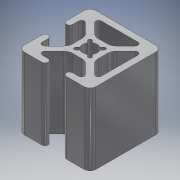
# Autodesk Inventor part: 1002-S
Saved by Autodesk Inventor 2017 SP1 (Build 210196100, 196)
## iProperties
Created: 2016-09-13
Part Number: 1002-S
Material: 6105-T5
Description: 40 S SHORT SINGLE UNIBEARING ASSEMBLY ON 40-4040 X 75mm
Document SubType Name: Modeling
Designer: BRALEF
Density: 1 g/cm^3
Appearance: CLEAR ANODIZED
MATERIAL: 6061-T6
PART PRICE: 44.65
Author: BRALEF
Autodesk Inventor part; units mm, degrees
ref_plane "YZ Plane" through (0, 0, 0) normal (1, 0, 0) x (0, 1, 0)
ref_plane "XZ Plane" through (0, 0, 0) normal (0, 1, 0) x (-1, 0, 0)
ref_plane "XY Plane" through (0, 0, 0) normal (0, 0, 1) x (1, 0, 0)
sketch "Sketch1" plane through (0, 0, 0) normal (0, 1, 0) x (-1, 0, 0)
  arc A0 (-1.9692, 2.8605) -> (-2.8605, 1.9692) centre (-2.4696, 2.4696) ccw
  line L0 (-2.2319, 1.3405) -> (-2.8605, 1.9692)
  arc A1 (-2.2319, 1.3405) -> (-2.2319, -1.3405) centre (0, 0) ccw
  line L1 (-2.8605, -1.9692) -> (-2.2319, -1.3405)
  arc A2 (-2.8605, -1.9692) -> (-1.9692, -2.8605) centre (-2.4696, -2.4696) ccw
  line L2 (-1.3405, -2.2319) -> (-1.9692, -2.8605)
  arc A3 (-1.3405, -2.2319) -> (1.3405, -2.2319) centre (0, 0) ccw
  line L3 (1.9692, -2.8605) -> (1.3405, -2.2319)
  arc A4 (1.9692, -2.8605) -> (2.8605, -1.9692) centre (2.4696, -2.4696) ccw
  line L4 (2.2319, -1.3405) -> (2.8605, -1.9692)
  arc A5 (2.2319, -1.3405) -> (2.2319, 1.3405) centre (0, 0) ccw
  line L5 (2.8605, 1.9692) -> (2.2319, 1.3405)
  arc A6 (2.8605, 1.9692) -> (1.9692, 2.8605) centre (2.4696, 2.4696) ccw
  line L6 (1.3405, 2.2319) -> (1.9692, 2.8605)
  arc A7 (1.3405, 2.2319) -> (-1.3405, 2.2319) centre (0, 0) ccw
  line L7 (-1.9692, 2.8605) -> (-1.3405, 2.2319)
  arc A8 (-8.7558, 7.1932) -> (-10.4902, 6.4748) centre (-9.4742, 6.4748) ccw
  line L8 (-10.4902, -6.4748) -> (-10.4902, 6.4748)
  arc A9 (-10.4902, -6.4748) -> (-8.7558, -7.1932) centre (-9.4742, -6.4748) ccw
  line L9 (-5.4471, -3.8845) -> (-8.7558, -7.1932)
  arc A10 (-5.4471, -3.8845) -> (-4.5172, -1.6395) centre (-7.6922, -1.6395) ccw
  line L10 (-4.5172, 1.6395) -> (-4.5172, -1.6395)
  arc A11 (-4.5172, 1.6395) -> (-5.4471, 3.8845) centre (-7.6922, 1.6395) ccw
  line L11 (-8.7558, 7.1932) -> (-5.4471, 3.8845)
  arc A12 (3.8845, -5.4471) -> (1.6395, -4.5172) centre (1.6395, -7.6922) ccw
  line L12 (-1.6395, -4.5172) -> (1.6395, -4.5172)
  arc A13 (-1.6395, -4.5172) -> (-3.8845, -5.4471) centre (-1.6395, -7.6922) ccw
  line L13 (-7.1932, -8.7558) -> (-3.8845, -5.4471)
  arc A14 (-7.1932, -8.7558) -> (-6.4748, -10.4902) centre (-6.4748, -9.4742) ccw
  line L14 (6.4748, -10.4902) -> (-6.4748, -10.4902)
  arc A15 (6.4748, -10.4902) -> (7.1932, -8.7558) centre (6.4748, -9.4742) ccw
  line L15 (3.8845, -5.4471) -> (7.1932, -8.7558)
  arc A16 (-12.7002, -10.5921) -> (-10.592, -12.7003) centre (-10.592, -10.5921) ccw
  line L16 (-12.7002, -10.5921) -> (-12.7002, 10.5915)
  arc A17 (-10.592, 12.6997) -> (-12.7002, 10.5915) centre (-10.592, 10.5915) ccw
  line L17 (-10.592, 12.6997) -> (-4.3561, 12.6997)
  arc A18 (-4.3561, 10.4899) -> (-4.3561, 12.6997) centre (-4.3561, 11.5948) ccw
  line L18 (-4.3561, 10.4899) -> (-6.4746, 10.4899)
  arc A19 (-6.4746, 10.4899) -> (-7.193, 8.7555) centre (-6.4746, 9.4739) ccw
  line L19 (-7.193, 8.7555) -> (-3.8847, 5.4472)
  arc A20 (-3.8847, 5.4472) -> (-1.6396, 4.5172) centre (-1.6396, 7.6922) ccw
  line L20 (-1.6396, 4.5172) -> (1.6395, 4.5172)
  arc A21 (1.6395, 4.5172) -> (3.8846, 5.4472) centre (1.6395, 7.6922) ccw
  line L21 (3.8846, 5.4472) -> (7.1929, 8.7555)
  arc A22 (7.1929, 8.7555) -> (6.4745, 10.4899) centre (6.4745, 9.4739) ccw
  line L22 (6.4745, 10.4899) -> (4.3561, 10.4899)
  arc A23 (4.3561, 12.6997) -> (4.3561, 10.4899) centre (4.3561, 11.5948) ccw
  line L23 (4.3561, 12.6997) -> (10.592, 12.6997)
  arc A24 (12.7002, 10.5915) -> (10.592, 12.6997) centre (10.592, 10.5915) ccw
  line L24 (12.7002, 10.5915) -> (12.7002, 4.3561)
  arc A25 (10.4904, 4.3561) -> (12.7002, 4.3561) centre (11.5953, 4.3561) ccw
  line L25 (10.4904, 4.3561) -> (10.4904, 6.475)
  arc A26 (10.4904, 6.475) -> (8.756, 7.1934) centre (9.4744, 6.475) ccw
  line L26 (8.756, 7.1934) -> (5.4472, 3.8846)
  arc A27 (5.4472, 3.8846) -> (4.5172, 1.6395) centre (7.6922, 1.6395) ccw
  line L27 (4.5172, 1.6395) -> (4.5172, -1.6396)
  arc A28 (4.5172, -1.6396) -> (5.4472, -3.8847) centre (7.6922, -1.6396) ccw
  line L28 (5.4472, -3.8847) -> (8.756, -7.1935)
  arc A29 (8.756, -7.1935) -> (10.4904, -6.4751) centre (9.4744, -6.4751) ccw
  line L29 (10.4904, -6.4751) -> (10.4904, -4.3561)
  arc A30 (12.7002, -4.3561) -> (10.4904, -4.3561) centre (11.5953, -4.3561) ccw
  line L30 (12.7002, -4.3561) -> (12.7002, -10.5921)
  arc A31 (10.592, -12.7003) -> (12.7002, -10.5921) centre (10.592, -10.5921) ccw
  line L31 (10.592, -12.7003) -> (-10.592, -12.7003)
  point P0 (0, 0)
  dimension "d23" = 8.183
  dimension "d69" = 1.016
  dimension "d70" = 3.175
  dimension "d86" = 17.2174
  dimension "d87" = 23.1904
  dimension "d88" = 25.4004
  dimension "d89" = 17.2169
  dimension "d90" = 23.1899
  dimension "d92" = 8.1825
  dimension "d93" = 2.2098
  dimension "d96" = 2.2097
  constraints: 64 end point, 64 point on circle, 64 tangent, 32 centre point, 21 equal radius, 16 parallel, 1 horizontal, 1 perpendicular, 1 vertical
  measures "d23" distance between parallel lines of L24 L27
  measures "d69" radius of A26
  measures "d70" radius of A27
  measures "d86" distance between parallel lines of L24 L10
  measures "d87" distance between parallel lines of L24 L8
  measures "d88" distance between parallel lines of L16 L24
  measures "d89" distance between parallel lines of L23 L12
  measures "d90" distance between parallel lines of L23 L14
  measures "d92" distance between parallel lines of L23 L20
  measures "d93" distance between parallel lines of L26 L21
  measures "d96" distance between parallel lines of L28 L15
extrude "Extrusion1" add sketch "Sketch1" along normal mid plane 25.4
body "Solid1"
